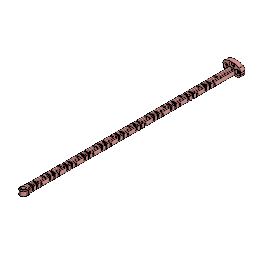
FlexpodV1 (Autodesk Fusion 360 archive; units mm, degrees)
design "FlexPod Leg"
Autodesk Fusion 360 part; units mm, degrees
other "DerivedContext1"
sketch "Sketch1" plane through (0, 0, 0) normal (0, 1, 0) x (1, 0, 0)
  circle A0 centre (0, 0) radius 2.9
  line L0 (3.9674, -4) -> (-3.9674, -4)
  line L1 (-3.9674, -4) -> (-3.9674, 4)
  line L2 (-3.9674, 4) -> (3.9674, 4)
  line L3 (3.9674, 4) -> (3.9674, -4)
  line L4 (3.9674, -4) -> (-3.9674, 4) construction
  line L5 (-3.9674, -4) -> (3.9674, 4) construction
  line L6 (-2.0422, -2.059) -> (-0.9, -3.1919)
  line L7 (-0.9, -3.1919) -> (0.9, -3.1919)
  line L8 (2.0422, -2.059) -> (0.9, -3.1919)
  line L9 (-2.0422, 2.059) -> (-0.9, 3.1919)
  line L10 (-0.9, 3.1919) -> (0.9, 3.1919)
  line L11 (2.0422, 2.059) -> (0.9, 3.1919)
  constraint coincident A0.centre origin
  constraint horizontal L0
  constraint perpendicular L0 L1
  constraint parallel L0 L2
  constraint parallel L1 L3
  constraint coincident L4 A0.centre
  constraint coincident L5 A0.centre
  constraint coincident A0 L6.start
  constraint coincident L5 L6.start
  constraint tangent A0 L6
  constraint horizontal L7
  constraint coincident A0 L8.start
  constraint coincident L4 L8.start
  constraint tangent A0 L8
  constraint coincident A0 L9.start
  constraint coincident L4 L9.start
  constraint tangent A0 L9
  constraint horizontal L10
  constraint coincident L5 L11.start
  constraint coincident A0 L11.start
  constraint coincident L10 L11.end
  constraint tangent A0 L11
  constraint equal L7 L10
  measures "d1" diameter of A0
  measures "d25" distance of L0.start L2.end
  measures "d30" distance of L6.end L7.end
extrude "Extrude1" add sketch "Sketch1" along normal blind 300
extrude "Extrude2" add sketch "Sketch1" along normal blind 10 contours A0 | A0 L9 L10 L11 | A0 L6 L7 L8
sketch "Sketch2" plane through (0, 300, 0) normal (0, 1, 0) x (-1, 0, 0)
  line L0 (-3.9674, -4) -> (3.9674, -4)
  line L1 (3.9674, -4) -> (3.9674, 4)
  line L2 (3.9674, 4) -> (-3.9674, 4)
  line L3 (-3.9674, 4) -> (-3.9674, -4)
  line L4 (12.5, 12.5) -> (-12.5, 12.5)
  line L5 (-12.5, 12.5) -> (-12.5, -12.5)
  line L6 (-12.5, -12.5) -> (12.5, -12.5)
  line L7 (12.5, -12.5) -> (12.5, 12.5)
  line L8 (12.5, 12.5) -> (-12.5, -12.5) construction
  line L9 (-12.5, 12.5) -> (12.5, -12.5) construction
  line L10 (-12.5, 0) -> (12.5, 0)
  line L11 (-12.5, -4) -> (12.5, -4)
  arc A0 (12.5, -4) -> (-12.5, -4) centre (0, -4) ccw
  line L12 (0, -9) -> (17.3205, 1)
  line L13 (0, -9) -> (-17.3205, 1)
  circle A1 centre (0, -9) radius 20
  arc A2 (-2.0422, 2.059) -> (-2.0422, -2.059) centre (0, 0) ccw
  line L14 (-2.0422, 2.059) -> (-0.9, 3.1919)
  line L15 (-0.9, 3.1919) -> (0.9, 3.1919)
  line L16 (0.9, 3.1919) -> (2.0422, 2.059)
  arc A3 (2.0422, -2.059) -> (2.0422, 2.059) centre (0, 0) ccw
  line L17 (2.0422, -2.059) -> (0.9, -3.1919)
  line L18 (0.9, -3.1919) -> (-0.9, -3.1919)
  line L19 (-0.9, -3.1919) -> (-2.0422, -2.059)
  dimension "d6" = 25
  dimension "d7" = 25
  constraint horizontal L4
  constraint perpendicular L4 L5
  constraint parallel L4 L6
  constraint parallel L5 L7
  constraint coincident L8 A2.centre
  constraint coincident L9 A2.centre
  constraint coincident A2.centre A3.centre
  constraint midpoint L5 L10.start
  constraint midpoint L7 L10.end
  constraint coincident L5 L11.start
  constraint coincident L7 L11.end
  constraint perpendicular L7 L11
  constraint tangent L7 A0
  constraint midpoint L0 A0.centre
  measures "d6" distance of L5.end L6.end
  measures "d7" distance of L4.end L5.end
extrude "Extrude3" add sketch "Sketch2" against normal blind 6 contours L3 L10 L11 A0 L13 | L1 L10 L11 A0 L12 | L1 L2 L3 L10 A0 | L5 L10 A0 L13 | L5 L7 L10 A0 A1 | L7 L10 A0 L12
sketch "Sketch3" plane through (0, 294, 0) normal (0, -1, 0) x (1, 0, 0)
  line L0 (3.9674, -4) -> (8.6603, -4)
  line L1 (-3.9674, -4) -> (-3.9674, 4)
  line L2 (-3.9674, 4) -> (3.9674, 4)
  line L3 (3.9674, 4) -> (3.9674, -4)
  line L4 (8.6603, -4) -> (12.5, -1.7831)
  line L5 (12.5, -1.7831) -> (12.5, 6.6125)
  arc A0 (12.5, 6.6125) -> (-12.5, 6.6125) centre (0, -9) ccw
  line L6 (-12.5, 6.6125) -> (-12.5, -1.7831)
  circle A1 centre (8, 2) radius 2
  circle A2 centre (0, 7.5) radius 2
  circle A3 centre (-8, 2) radius 2
  line L7 (-12.5, -1.7831) -> (-8.6603, -4)
  line L8 (9.6291, 3.1602) -> (8.875, 4.2191)
  line L9 (8.875, 4.2191) -> (7.125, 4.2191)
  line L10 (7.125, 4.2191) -> (6.3709, 3.1602)
  line L11 (1.6291, 8.6602) -> (0.875, 9.7191)
  line L12 (0.875, 9.7191) -> (-0.875, 9.7191)
  line L13 (-0.875, 9.7191) -> (-1.6291, 8.6602)
  line L14 (-6.3709, 3.1602) -> (-7.125, 4.2191)
  line L15 (-7.125, 4.2191) -> (-8.875, 4.2191)
  line L16 (-8.875, 4.2191) -> (-9.6291, 3.1602)
  line L17 (9.6291, 0.8398) -> (8.875, -0.2191)
  line L18 (8.875, -0.2191) -> (7.125, -0.2191)
  line L19 (7.125, -0.2191) -> (6.3709, 0.8398)
  line L20 (1.6291, 6.3398) -> (0.875, 5.2809)
  line L21 (0.875, 5.2809) -> (-0.875, 5.2809)
  line L22 (-0.875, 5.2809) -> (-1.6291, 6.3398)
  line L23 (-6.3709, 0.8398) -> (-7.125, -0.2191)
  line L24 (-7.125, -0.2191) -> (-8.875, -0.2191)
  line L25 (-8.875, -0.2191) -> (-9.6291, 0.8398)
  line L26 (-8.6603, -4) -> (-3.9674, -4)
  dimension "d13" = 4
  dimension "d14" = 4
  dimension "d15" = 4
  dimension "d71" = 1.75
  constraint coincident A1 L8.start
  constraint horizontal L9
  constraint coincident A1 L10.end
  constraint coincident A2 L11.start
  constraint tangent A2 L11
  constraint horizontal L12
  constraint coincident A2 L13.end
  constraint coincident A3 L14.start
  constraint parallel L12 L15
  constraint coincident A3 L16.end
  constraint equal L14 L16
  constraint tangent A2 L13
  constraint tangent A1 L10
  constraint tangent A1 L8
  constraint equal L8 L10
  constraint equal L11 L13
  constraint equal L9 L12
  constraint equal L12 L15
  constraint tangent A3 L16
  constraint tangent A3 L14
  constraint equal L10 L14
  constraint equal L10 L11
  constraint coincident A1 L17.start
  constraint horizontal L18
  constraint coincident A1 L19.end
  constraint tangent A1 L19
  constraint coincident A2 L20.start
  constraint parallel L2 L21
  constraint coincident A2 L22.end
  constraint tangent A2 L22
  constraint coincident A3 L23.start
  constraint parallel L2 L24
  constraint coincident A3 L25.end
  constraint tangent A3 L25
  constraint equal L16 L25
  constraint equal L15 L24
  constraint equal L14 L23
  constraint tangent A3 L23
  constraint tangent A1 L17
  constraint tangent A2 L20
  constraint equal L10 L19
  constraint equal L8 L17
  constraint equal L9 L18
  constraint equal L13 L22
  constraint equal L11 L20
  constraint equal L12 L21
  measures "d13" diameter of A1
  measures "d14" diameter of A2
  measures "d15" diameter of A3
  measures "d71" distance of L8.end L9.end
extrude "Extrude4" cut sketch "Sketch3" against normal blind 8 contours A1 | A2 | A3
chamfer "Chamfer2" distance 1.5 angle 45 3 edges at (6.1353, 294, 2.7232) (-1.8647, 294, 8.2232) (-9.8647, 294, 2.7232)
extrude "Extrude11" cut sketch "Sketch3" against normal blind 15 contours A1 L8 L9 L10 | A1 L17 L18 L19 | A2 L11 L12 L13 | A2 L20 L21 L22 | A3 L14 L15 L16 | A3 L23 L24 L25
sketch "Sketch4" plane through (0, 0, 4) normal (0, 0, 1) x (-1, 0, 0)
  line L0 (-3.9674, -294) -> (0, -294)
  line L1 (3.9674, -294) -> (3.9674, 0)
  line L2 (3.9674, 0) -> (-3.9674, 0)
  line L3 (-3.9674, 0) -> (-3.9674, -294)
  circle A0 centre (0, -5) radius 2.6
  line L4 (5, 0) -> (-5, 0)
  line L5 (-5, 0) -> (-5, -10)
  line L6 (-5, -10) -> (5, -10)
  line L7 (5, -10) -> (5, 0)
  line L8 (5, 0) -> (-5, -10) construction
  line L9 (-5, 0) -> (5, -10) construction
  line L10 (0, -294) -> (3.9674, -294)
  point P0 (0, -5)
  dimension "d19" = 5.2
  constraint horizontal L4
  constraint perpendicular L4 L5
  constraint parallel L4 L6
  constraint parallel L5 L7
  constraint coincident L8 P0
  constraint coincident L9 P0
  constraint coincident P0 A0.centre
  measures "d19" diameter of A0
extrude "Extrude5" cut sketch "Sketch4" against normal blind 17 contours A0
extrude "Extrude6" add sketch "Sketch4" against normal blind 8 contours L3 L4 L5 L6 | L1 L4 L6 L7
fillet "Fillet2" radius 5 4 edges at (-5, 0, 0) (-5, 10, 0) (5, 10, 0) (5, 0, 0)
chamfer "Chamfer4" distance 1 angle 45 16 edges at (4.7348, 8.5637, -4) (5, 5.9785, -4) (3.5355, 1.4645, -4) (-3.5355, 1.4645, -4) (-5, 5.9785, -4) (-4.7348, 8.5637, -4) (3.9674, 152, -4) (-3.9674, 152, -4) (3.9674, 152, 4) (-3.9674, 152, 4) (3.5355, 1.4645, 4) (-3.5355, 1.4645, 4) (-5, 5.9785, 4) (-4.7348, 8.5637, 4) (4.7348, 8.5637, 4) (5, 5.9785, 4)
sketch "Sketch5" plane through (0, 0, 4) normal (0, 0, 1) x (-1, 0, 0)
  line L0 (-2.9674, -294) -> (0, -294)
  line L1 (5, -15) -> (-5, -15)
  line L2 (-5, -15) -> (-5, -13)
  line L3 (-5, -13) -> (5, -13)
  line L4 (5, -13) -> (5, -15)
  line L5 (5, -25) -> (-5, -25)
  line L6 (-5, -25) -> (-5, -27)
  line L7 (-5, -27) -> (5, -27)
  line L8 (5, -27) -> (5, -25)
  line L9 (2.9674, -294) -> (2.9674, -9.6393)
  line L10 (-2.9674, -9.6393) -> (-2.9674, -294)
  line L11 (0, -294) -> (2.9674, -294)
  dimension "d35" = 2
  dimension "d36" = 10
  constraint horizontal L1
  constraint vertical L2
  constraint horizontal L3
  constraint vertical L4
  constraint horizontal L5
  constraint vertical L6
  constraint horizontal L7
  constraint vertical L8
  measures "d35" distance of L5.end L6.end
  measures "d36" distance of L1 L5
extrude "Extrude7" cut sketch "Sketch5" against normal blind 5 contours L1 L3 L9 L10 | L1 L2 L3 L10 | L1 L3 L4 L9
extrude "Extrude8" cut sketch "Sketch5" along normal blind 5 from surface at -8 contours L5 L7 L9 L10 | L5 L6 L7 L10 | L5 L7 L8 L9
sketch "Sketch6" plane through (3.9674, 0, 0) normal (1, 0, 0) x (0, 1, 0)
  line L0 (27, 1) -> (27, -3)
  line L1 (294, -3) -> (294, 3)
  line L2 (15, 3) -> (15, -1)
  line L3 (15, -1) -> (13, -1)
  line L4 (13, -1) -> (13, 3)
  line L5 (10, 3) -> (10, -3)
  line L6 (25, -3) -> (25, 1)
  line L7 (25, 1) -> (27, 1)
  line L8 (15, 3) -> (15, -1)
  line L9 (25, -3) -> (25, 1)
  line L10 (19, 5) -> (21, 5)
  line L11 (21, 5) -> (21, -5)
  line L12 (21, -5) -> (19, -5)
  line L13 (19, -5) -> (19, 5)
  line L14 (31, 5) -> (33, 5)
  line L15 (33, 5) -> (33, -5)
  line L16 (33, -5) -> (31, -5)
  line L17 (31, -5) -> (31, 5)
  line L18 (27, 1) -> (27, -3)
  line L19 (27, -3) -> (294, -3)
  line L20 (294, 3) -> (15, 3)
  line L21 (13, 3) -> (10, 3)
  line L22 (10, -3) -> (25, -3)
  dimension "d40" = 2
  dimension "d43" = 10
  dimension "d44" = 4
  constraint horizontal L10
  constraint vertical L11
  constraint horizontal L12
  constraint vertical L13
  constraint horizontal L14
  constraint vertical L15
  constraint horizontal L16
  constraint vertical L17
  measures "d40" distance of L11.end L12.end
  measures "d43" distance of L11 L17
  measures "d44" distance of L9 L11
extrude "Extrude9" cut sketch "Sketch6" against normal blind 5 contours L11 L13 L20 L22 | L11 L12 L13 L22 | L10 L11 L13 L20
extrude "Extrude10" cut sketch "Sketch6" along normal blind 5 from surface at -7.9349 contours L15 L16 L17 L19 | L15 L17 L19 L20 | L14 L15 L17 L20
chamfer "Chamfer5" distance 0.75 angle 45 8 edges at (-2.9, 300, 0) (-1.4711, 300, -2.6254) (-1.4711, 300, 2.6254) (1.4711, 300, -2.6254) (2.9, 300, 0) (1.4711, 300, 2.6254) (0, 300, -3.1919) (0, 300, 3.1919)
fillet "Fillet3" radius 5 4 edges at (12.5, 297, -1.7831) (-12.5, 297, -1.7831) (12.5, 297, 6.6125) (-12.5, 297, 6.6125)
pattern_linear "R-Pattern2" count 11 spacing 24 along (0, 1, 0) of "Extrude7"
pattern_linear "R-Pattern3" count 11 spacing 24 along (0, 1, 0) of "Extrude8"
pattern_linear "R-Pattern4" count 11 spacing 24 along (0, 1, 0) of "Extrude9"
pattern_linear "R-Pattern5" count 11 spacing 24 along (0, 1, 0) of "Extrude10"
